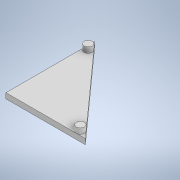
# Autodesk Inventor part: 零件2
Saved by Autodesk Inventor 2022 (Build 260153000, 153)
## iProperties
Created: 2023-03-09
Part Number: 零件2
Material: 一般
Document SubType Name: Modeling
Designer: JOU
Density: 1 g/cm^3
Appearance: 預設
Author: JOU
Autodesk Inventor part; units mm, degrees
ref_plane "YZ Plane" through (0, 0, 0) normal (1, 0, 0) x (0, 1, 0)
ref_plane "XZ Plane" through (0, 0, 0) normal (0, 1, 0) x (-1, 0, 0)
ref_plane "XY Plane" through (0, 0, 0) normal (0, 0, 1) x (1, 0, 0)
sketch "草圖1" plane through (0, 0, 0) normal (0, 1, 0) x (-1, 0, 0)
  line L0 (0, 0) -> (14.7102, 0)
  line L1 (14.7102, 0) -> (14.7102, -16.4216)
  line L2 (14.7102, -16.4216) -> (0, 0)
  constraints: 6 end point, 1 horizontal, 1 perpendicular
extrude "擠出1" add sketch "草圖1" along normal blind 1
sketch "草圖2" plane through (0, 1, 0) normal (0, 1, 0) x (1, 0, 0)
  circle A0 centre (-13.9602, 14.4603) radius 0.75
  line L0 (-14.7102, 16.4216) -> (-14.7102, 0) projected
  line L1 (0, 0) -> (-14.7102, 16.4216) projected
  dimension "d2" = 1.5
  constraints: 2 tangent, 1 centre point
  measures "d2" diameter of A0
extrude "擠出2" add sketch "草圖2" along normal blind 1 contours A0
sketch "草圖3" plane through (0, 1, 0) normal (0, 1, 0) x (1, 0, 0)
  circle A0 centre (-1.6787, 0.75) radius 0.75
  circle A1 centre (-13.9602, 14.4603) radius 0.75 projected
  line L0 (-14.7102, 0) -> (0, 0) projected
  line L1 (0, 0) -> (-13.4016, 14.9607) projected
  constraints: 2 tangent, 1 centre point, 2 other
extrude "擠出3" add sketch "草圖3" along normal up to surface (1 mm away) contours A0
